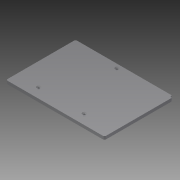
# Autodesk Inventor part: zCarPlexiBed
Saved by Autodesk Inventor 2013 (Build 170138000, 138)
## iProperties
Created: 2015-01-14
Part Number: zCarPlexiBed
Material: Generic
Document SubType Name: Modeling
Designer: dzban
Density: 1 g/cm^3
Author: dzban
Autodesk Inventor part; units mm, degrees
ref_plane "YZ Plane" through (0, 0, 0) normal (1, 0, 0) x (0, 1, 0)
ref_plane "XZ Plane" through (0, 0, 0) normal (0, 1, 0) x (-1, 0, 0)
ref_plane "XY Plane" through (0, 0, 0) normal (0, 0, 1) x (1, 0, 0)
sketch "Sketch1" plane through (0, 0, 0) normal (0, 0, 1) x (1, 0, 0)
  circle A0 centre (-79, 26.5) radius 2.5
  circle A1 centre (-198, 26.5) radius 2.5
  circle A2 centre (-138.5, 171.5) radius 2.5
  line L0 (-4, 0) -> (-253, 0)
  arc A3 (-4, 0) -> (0, 4) centre (-4, 4) ccw
  line L1 (0, 174.5) -> (0, 4)
  arc A4 (0, 174.5) -> (-2, 176.5) centre (-2, 174.5) ccw
  line L2 (-3, 176.5) -> (-2, 176.5)
  arc A5 (-5, 178.5) -> (-3, 176.5) centre (-3, 178.5) ccw
  line L3 (-5, 179.5) -> (-5, 178.5)
  arc A6 (-5, 179.5) -> (-7, 181.5) centre (-7, 179.5) ccw
  line L4 (-253, 181.5) -> (-7, 181.5)
  arc A7 (-253, 181.5) -> (-257, 177.5) centre (-253, 177.5) ccw
  line L5 (-257, 4) -> (-257, 177.5)
  arc A8 (-257, 4) -> (-253, 0) centre (-253, 4) ccw
  point P0 (0, 0)
  point P1 (0, 0)
  dimension "d2" = 119
  dimension "d4" = 145
  dimension "d5" = 59.5
  dimension "d6" = 79
  dimension "d7" = 26.5
  dimension "d8" = 10
  dimension "d9" = 59
  dimension "d10" = 5
  dimension "d11" = 5
  dimension "d12" = 5
  dimension "d13" = 4
  dimension "d14" = 2
  dimension "d15" = 2
  dimension "d16" = 4
  dimension "d17" = 4
  dimension "d18" = 5
  dimension "d19" = 5
  constraints: 12 end point, 12 point on circle, 11 tangent, 9 centre point, 2 horizontal, 2 horizontal alignment, 2 vertical, 1 vertical alignment
  measures "d2" distance of A0.centre A1.centre
  measures "d4" vertical distance of A2.centre A0.centre
  measures "d5" horizontal distance of A2.centre A0.centre
  measures "d6" distance from line of L1 A0.centre
  measures "d7" distance from line of A0.centre L0
  measures "d8" distance from line of L4 A2.centre
  measures "d9" distance from line of L5 A1.centre
  measures "d10" diameter of A1
  measures "d11" diameter of A0
  measures "d12" diameter of A2
  measures "d13" radius of A8
  measures "d14" radius of A6
  measures "d15" radius of A4
  measures "d16" radius of A7
  measures "d17" radius of A3
  measures "d18" distance between parallel lines of L4 L2
  measures "d19" distance between parallel lines of L1 L3
extrude "Extrusion1" add sketch "Sketch1" along normal blind 8
sketch "Sketch3" plane through (0, 0, 8) normal (0, 0, 1) x (1, 0, 0)
  circle A0 centre (-79, 26.5) radius 2.5 projected
  circle A1 centre (-198, 26.5) radius 2.5 projected
  circle A2 centre (-138.5, 171.5) radius 2.5 projected
  point P0 (0, 0)
hole "Hole1" at (-198, 26.5, 8) at (-79, 26.5, 8) at (-138.5, 171.5, 8) direction (0, 0, -1) diameter 10 depth 0 tip angle 91
body "Solid1"
